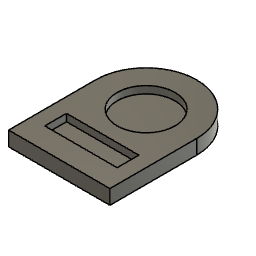
EX1 (Autodesk Fusion 360 design; units mm, degrees)
Autodesk Fusion 360 part; units mm, degrees
sketch "Sketch1" plane through (0, 0, 0) normal (0, 1, 0) x (1, 0, 0)
  line L0 (0, 0) -> (70, 0)
  line L1 (70, 0) -> (70, 60)
  line L2 (0, 60) -> (0, 0)
  arc A0 (70, 60) -> (0, 60) centre (35, 60) ccw
  line L3 (60, 30) -> (10, 30)
  line L4 (10, 30) -> (10, 15)
  line L5 (10, 15) -> (60, 15)
  line L6 (60, 15) -> (60, 30)
  arc A1 (15, 60) -> (55, 60) centre (35, 60) ccw
  arc A2 (55, 60) -> (15, 60) centre (35, 60) ccw
  point P0 (35, 22.5)
  dimension "d1" = 70
  dimension "d2" = 60
  dimension "d5" = 50
  dimension "d6" = 15
  dimension "d7" = 15
  dimension "d8" = 10
  dimension "d10" = 35
  dimension "d11" = 20
  constraint horizontal L0
  constraint vertical L1
  constraint vertical L2
  constraint coincident L0.start L2.end
  constraint horizontal L3
  constraint perpendicular L3 L4
  constraint parallel L3 L5
  constraint parallel L4 L6
  constraint concentric A1 A2
  measures "d1" distance of L0.start L0.end
  measures "d2" distance of L0.start L2.start
  measures "d5" distance of L4.end L5.end
  measures "d6" distance of L3.end L4.end
  measures "d7" distance of L0 L5
  measures "d8" distance of L2 L4
  measures "d10" radius of A0
  measures "d11" radius of A2
extrude "Extrude1" add sketch "Sketch1" along normal blind 10
extrude "Extrude2" add sketch "Sketch1" along normal blind 5 contours L3 L4 L5 L6 | A1 A2
